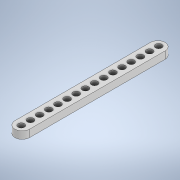
# Autodesk Inventor part: rearLeg_bot
Saved by Autodesk Inventor 2020 (Build 240168000, 168)
## iProperties
Created: 2019-04-04
Part Number: rearLeg_bot
Material: Generic
Document SubType Name: Modeling
Designer: mfans
Density: 1 g/cm^3
Appearance: Default
Author: mfans
Autodesk Inventor part; units mm, degrees
ref_plane "YZ Plane" through (0, 0, 0) normal (1, 0, 0) x (0, 1, 0)
ref_plane "XZ Plane" through (0, 0, 0) normal (0, 1, 0) x (-1, 0, 0)
ref_plane "XY Plane" through (0, 0, 0) normal (0, 0, 1) x (1, 0, 0)
sketch "Sketch1" plane through (0, 0, 0) normal (0, 1, 0) x (-1, 0, 0)
  line L0 (4, 40) -> (-4, 40)
  line L1 (-4, 40) -> (-4, -40)
  line L2 (-4, -40) -> (4, -40)
  line L3 (4, -40) -> (4, 40)
  line L4 (4, 40) -> (-4, -40) construction
  line L5 (-4, 40) -> (4, -40) construction
  point P0 (0, 0)
  dimension "d0" = 8
  dimension "d1" = 80
  constraints: 12 end point, 2 midpoint, 2 parallel, 1 horizontal, 1 perpendicular
  measures "d0" distance of L1.end L2.end
  measures "d1" distance of L0.end L1.end
extrude "Extrusion1" add sketch "Sketch1" along normal blind 4
sketch "Sketch2" plane through (0, 4, 0) normal (0, 1, 0) x (1, 0, 0)
  line L0 (-4, -40) -> (4, -40) projected
  line L1 (-4, 40) -> (-4, -40) projected
  line L2 (-4, -40) -> (4, -40) projected
  line L3 (4, -40) -> (4, 40) projected
  line L4 (4, 40) -> (-4, 40) projected
  point P0 (0, 0)
  point P1 (0, -37.5)
  point P2 (0, -32.5)
  point P3 (0, -27.5)
  point P4 (0, -22.5)
  point P5 (0, -17.5)
  point P6 (0, -12.5)
  point P7 (0, -7.5)
  point P8 (0, -2.5)
  point P9 (0, 2.5)
  point P10 (0, 7.5)
  point P11 (0, 12.5)
  point P12 (0, 17.5)
  point P13 (0, 22.5)
  point P14 (0, 27.5)
  point P15 (0, 32.5)
  point P16 (0, 37.5)
  dimension "d4" = 2.5
  dimension "d7" = 5
  constraints: 1 vertical, 15 other
  measures "d4" distance from line of L0 point (0, -37.5)
  measures "d7" distance of point (0, -37.5) point (0, -32.5)
hole "Hole1" at (0, 4, 37.5) at (0, 4, 32.5) at (0, 4, 27.5) at (0, 4, 22.5) at (0, 4, 17.5) at (0, 4, 12.5) at (0, 4, 7.5) at (0, 4, 2.5) at (0, 4, -2.5) at (0, 4, -7.5) at (0, 4, -12.5) at (0, 4, -17.5) at (0, 4, -22.5) at (0, 4, -27.5) at (0, 4, -32.5) at (0, 4, -37.5) direction (0, -1, 0) diameter 3.5 end through all
thicken "Thicken1" operation add thickness 1 both sides no extend neighbours yes toward (0, 0, 1) faces at (-1.3333, 1.3333, 40)
thicken "Thicken2" operation add thickness 1 both sides no extend neighbours yes toward (0, 0, -1) faces at (1.3333, 1.3333, -40)
fillet "Fillet1" radius 4 4 edges at (-4, 2, -41) (4, 2, -41) (4, 2, 41) (-4, 2, 41)
body "Solid1"
